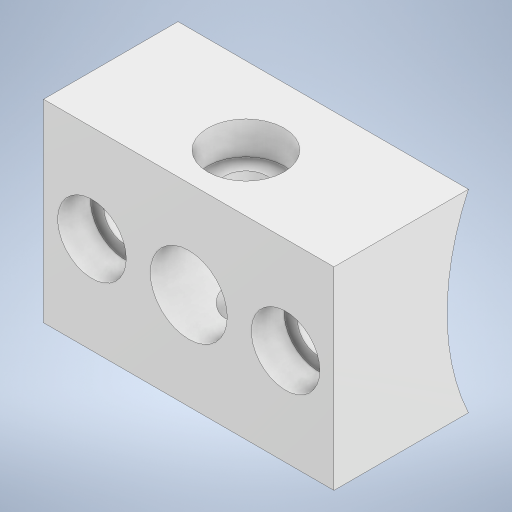
# Autodesk Inventor part: Axial Holder
Saved by Autodesk Inventor 2023 (Build 270158030, 158C)
## iProperties
Created: 2022-10-03
Part Number: Axial Holder
Material: ABS Plastic
Document SubType Name: Modeling
Designer: cjj5381
Density: 1.06 g/cm^3
Appearance: Smooth - White
Author: cjj5381
Autodesk Inventor part; units mm, degrees
ref_plane "YZ Plane" through (0, 0, 0) normal (1, 0, 0) x (0, 1, 0)
ref_plane "XZ Plane" through (0, 0, 0) normal (0, 1, 0) x (-1, 0, 0)
ref_plane "XY Plane" through (0, 0, 0) normal (0, 0, 1) x (1, 0, 0)
sketch "Sketch1" plane through (0, 0, 0) normal (1, 0, 0) x (0, 1, 0)
  arc A0 (12.7, -17.6415) -> (-12.7, -17.6415) centre (0, -45) ccw
  line L0 (0, 0) -> (0, -134.2841)
  line L1 (-12.7, 0) -> (-12.7, -17.6415)
  line L2 (12.7, -17.6415) -> (12.7, 0)
  line L3 (12.7, 0) -> (-12.7, 0)
  dimension "d0" = 60.325
  dimension "d47" = 45
  dimension "d48" = 25.4
  constraints: 8 end point, 2 point on circle, 1 centre point, 1 horizontal, 1 parallel, 1 point on line, 1 vertical, 1 other
  measures "d0" diameter of A0
  measures "d47" distance of L0.start A0.centre
  measures "d48" distance of L2.end L1.start
extrude "Extrusion1" add sketch "Sketch1" along normal blind 38.1
sketch "Sketch8" plane through (0, -12.7, 0) normal (0, 0, 1) x (1, 0, 0)
  circle A0 centre (19.05, 12.7) radius 5.05
  line L0 (0, 12.7) -> (38.1, 12.7) construction
  line L1 (0, 25.4) -> (38.1, 25.4) construction
  line L2 (38.1, 25.4) -> (38.1, 0) construction
  dimension "d49" = 10.1
  constraints: 2 end point, 2 midpoint, 1 centre point, 1 horizontal
  measures "d49" diameter of A0
extrude "Extrusion6" cut sketch "Sketch8" against normal through all
sketch "Sketch10" plane through (0, 12.7, 0) normal (0, 1, 0) x (1, 0, 0)
  line L0 (0, 17.6415) -> (0, 0) projected
  line L1 (0, 0) -> (38.1, 0) projected
  line L2 (19.05, 0) -> (19.05, 20.4763) construction
  point P0 (19.05, 7.5)
  dimension "d60" = 7.5
  constraints: 2 end point, 1 midpoint, 1 point on line, 1 vertical
  measures "d60" distance from line of L1 point (19.05, 7.5)
hole "Hole2" at (19.05, 12.7, -7.5) direction (0, -1, 0) diameter 5.5 end through all counterbore diameter 10 counterbore depth 4.3 clearance for "Hex Head Cap Screw ISO 24017" size "M5" standard "ISO"
sketch "Sketch11" plane through (0, -12.7, 0) normal (0, 0, 1) x (1, 0, 0)
  line L0 (0, 12.7) -> (38.1, 12.7) construction
  line L1 (38.1, 25.4) -> (38.1, 0) construction
  line L2 (0, 0) -> (38.1, 0) construction
  line L3 (19.05, 0) -> (19.05, 29.1053) construction
  point P0 (31.75, 12.7)
  point P1 (6.35, 12.7)
  dimension "d68" = 25.4
  constraints: 4 end point, 2 midpoint, 2 point on line, 1 symmetric about line, 1 vertical
  measures "d68" distance of point (6.35, 12.7) point (31.75, 12.7)
hole "Hole3" at (31.75, 0, 0) at (6.35, 0, 0) direction (0, 0, -1) diameter 5.5 end through all counterbore diameter 9 counterbore depth 4.3 clearance for "Hex Head Cap Screw ISO 24017" size "M5" standard "ISO"
body "Solid1"
